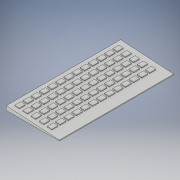
# Autodesk Inventor part: Slim_Keyboard
Saved by Autodesk Inventor 2019 (Build 230136000, 136)
## iProperties
Created: 2019-05-23
Part Number: Slim_Keyboard
Material: Generic
Document SubType Name: Modeling
Designer: Jorian Bruslind
Density: 1 g/cm^3
Appearance: Default
Author: Jorian Bruslind
Autodesk Inventor part; units mm, degrees
ref_plane "YZ Plane" through (0, 0, 0) normal (1, 0, 0) x (0, 1, 0)
ref_plane "XZ Plane" through (0, 0, 0) normal (0, 1, 0) x (-1, 0, 0)
ref_plane "XY Plane" through (0, 0, 0) normal (0, 0, 1) x (1, 0, 0)
sketch "Sketch1" plane through (0, 0, 0) normal (0, 1, 0) x (-1, 0, 0)
  line L0 (0, 0) -> (130, 0)
  line L1 (130, 0) -> (130, -280)
  line L2 (130, -280) -> (0, -280)
  line L3 (0, -280) -> (0, 0)
  dimension "d0" = 130
  dimension "d1" = 280
  constraints: 8 end point, 2 parallel, 1 horizontal, 1 perpendicular
  measures "d0" distance of L1.end L2.end
  measures "d1" distance of L0.end L1.end
extrude "Extrusion1" add sketch "Sketch1" along normal blind 10
sketch "Sketch2" plane through (-130, 0, 0) normal (0, 0, 1) x (1, 0, 0)
  line L0 (130, 0) -> (130, 2)
  line L1 (130, 0) -> (130, 10) projected
  line L2 (0, 10) -> (130, 10) projected
  line L3 (130, 2) -> (0, 10)
  line L4 (130, 2) -> (130, 10)
  line L5 (130, 10) -> (0, 10)
  dimension "d4" = 2
  constraints: 8 end point, 1 collinear, 1 perpendicular, 1 point on line
  measures "d4" distance of L0.start L0.end
extrude "Extrusion2" cut sketch "Sketch2" against normal up to next
sketch "Sketch3" plane through (-130, 10, 0) normal (0.0614223, 0.9981119, 0) x (0.9981119, -0.0614223, 0)
  line L0 (0.6142, 0) -> (0.6142, 280) projected
  line L1 (0.6142, 0) -> (0.6142, 10)
  line L2 (0.6142, 10) -> (10.6142, 10)
  line L3 (10.6142, 10) -> (21.6142, 10)
  line L4 (21.6142, 10) -> (21.6142, 25)
  line L5 (21.6142, 25) -> (10.6142, 25)
  line L6 (10.6142, 25) -> (10.6142, 10)
  point P0 (130.3688, 0)
  dimension "d7" = 10
  dimension "d8" = 10
  dimension "d9" = 11
  dimension "d10" = 15
  constraints: 12 end point, 2 parallel, 2 perpendicular, 1 horizontal, 1 point on line
  measures "d7" distance of L0.start L1.end
  measures "d8" distance of L1.end L2.end
  measures "d9" distance of L5.end L4.end
  measures "d10" distance of L4.end L3.end
extrude "Extrusion3" add sketch "Sketch3" along normal blind 2
pattern_linear "Rectangular Pattern1" count 13 spacing 20 along (0, 0, -1) count 5 spacing 20 along (0.9981119, -0.0614223, 0) of "Extrusion3"
body "Solid1"
